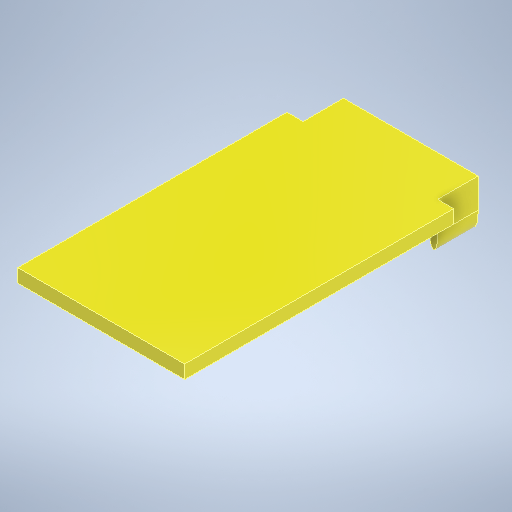
# Autodesk Inventor part: Soporte
Saved by Autodesk Inventor 2025.3 (Build 293356000, 356)
## iProperties
Created: 2025-09-16
Part Number: Soporte
Material: Generic
Document SubType Name: Modeling
Designer: steve
Density: 1 g/cm^3
Appearance: Yellow
Author: steve
Autodesk Inventor part; units mm, degrees
ref_plane "YZ Plane" through (0, 0, 0) normal (1, 0, 0) x (0, 1, 0)
ref_plane "XZ Plane" through (0, 0, 0) normal (0, 1, 0) x (-1, 0, 0)
ref_plane "XY Plane" through (0, 0, 0) normal (0, 0, 1) x (1, 0, 0)
sketch "Sketch1" plane through (0, 0, 0) normal (0, 0, 1) x (1, 0, 0)
  line L0 (-25, 0) -> (25, 0) construction
  line L1 (-25, 25.5) -> (-25, -25.5)
  line L2 (-28, 25.5) -> (-28, -25.5)
  line L3 (0, 25.5) -> (0, -25.5) construction
  line L4 (25, 25.5) -> (25, -25.5)
  line L5 (28, 25.5) -> (28, -25.5)
  line L6 (-25, -25.5) -> (-25, -19.5)
  line L7 (-25, 25.5) -> (-25, 19.5)
  line L8 (-25, 19.5) -> (-25, 26.8474) construction
  line L9 (-25, 26.8474) -> (-22.3693, 26.8474) construction
  line L10 (-22.3693, 26.8474) -> (-18.3013, 21.6592) construction
  spline S0 degree 3 poles (-25, 19.5) (-25, 26.8474) (-22.3693, 26.8474) (-18.3013, 21.6592) knots 1 1 1 1 2 2 2 2
  line L11 (25, 19.5) -> (25, 26.8474) construction
  line L12 (25, 26.8474) -> (22.3693, 26.8474) construction
  line L13 (22.3693, 26.8474) -> (18.3013, 21.6592) construction
  spline S1 degree 3 poles (25, 19.5) (25, 26.8474) (22.3693, 26.8474) (18.3013, 21.6592) knots 1 1 1 1 2 2 2 2
  arc A0 (18.3013, 21.6592) -> (-18.3013, 21.6592) centre (0, -20.023) ccw
  line L14 (-25, -19.5) -> (-25, -27.5122) construction
  line L15 (-25, -27.5122) -> (-22, -27.5122) construction
  line L16 (-22, -27.5122) -> (-22, -19.5) construction
  spline S2 degree 3 poles (-25, -19.5) (-25, -27.5122) (-22, -27.5122) (-22, -19.5) knots 1 1 1 1 2 2 2 2
  line L17 (25, -19.5) -> (25, -27.5122) construction
  line L18 (25, -27.5122) -> (22, -27.5122) construction
  line L19 (22, -27.5122) -> (22, -19.5) construction
  spline S3 degree 3 poles (25, -19.5) (25, -27.5122) (22, -27.5122) (22, -19.5) knots 1 1 1 1 2 2 2 2
  arc A1 (-22, -19.5) -> (22, -19.5) centre (0, 17.8333) ccw
  line L20 (-25, -25.5) -> (-25, -8.5)
  line L21 (-25, -8.5) -> (25, -8.5)
  line L22 (0, -25.5) -> (0, -13.5)
  line L23 (22, -13.5) -> (-22, -13.5)
  line L24 (-22, -19.5) -> (-22, -13.5)
  line L25 (22, -19.5) -> (22, -13.5)
  point P0 (0, 0)
  point P1 (-28, 0)
  point P2 (25, -19.5001)
  dimension "d0" = 50
  dimension "d1" = 3
  dimension "d2" = 51
  dimension "d3" = 3
  dimension "d4" = 51
  dimension "d5" = 51
  dimension "d6" = 0
  dimension "d7" = 6
  dimension "d10" = 6
  dimension "d11" = 3
  dimension "d12" = 17
  dimension "d13" = 12
  constraints: 28 end point, 8 symmetric about line, 7 point on line, 6 midpoint, 6 point on circle, 6 vertical, 2 centre point, 2 horizontal, 2 perpendicular, 1 parallel, 12 other
  measures "d0" distance of L0.start L0.end
  measures "d1" distance between parallel lines of L2 L1
  measures "d2" distance of L3.start L3.end
  measures "d3" distance between parallel lines of L4 L5
  measures "d4" distance of L1.start L1.end
  measures "d5" distance of L2.start L2.end
  measures "d6" vertical distance of point (-28, 0) L0.start
  measures "d7" distance of L1.end L6.end
  measures "d10" distance of L1.start L7.end
  measures "d11" distance of L6.end L16.end
  measures "d12" distance of L1.end L20.end
  measures "d13" distance of L3.end L22.end
extrude "Extrusion1" add sketch "Sketch1" along normal mid plane 15 contours L21 L4 S3 L25 L23 L24 S2 L1
sketch "Sketch3" plane through (0, 0, 7.5) normal (0, 0, 1) x (1, 0, 0)
  line L0 (-25, -8.5) -> (-25, -19.5) projected
  line L1 (25, -8.5) -> (-25, -8.5) projected
  line L2 (25, -19.5001) -> (25, -8.5) projected
  line L3 (-22, -13.5) -> (22, -13.5) projected
  line L4 (22, -13.5) -> (22, -19.5) projected
  line L5 (-22, -19.5) -> (-22, -13.5) projected
  line L6 (-25, -8.5) -> (25, -8.5)
  line L7 (-31, -8.5) -> (31, -8.5)
  line L8 (-31, -8.5) -> (-31, -13.5)
  line L9 (-31, -13.5) -> (31, -13.5)
  line L10 (31, -13.5) -> (31, -8.5)
  point P0 (0, 0)
  point P1 (0, -8.5)
  dimension "d17" = 62
  constraints: 10 end point, 2 midpoint, 2 point on line, 1 horizontal, 1 horizontal alignment, 1 parallel, 1 perpendicular, 1 other
  measures "d17" distance of L7.start L7.end
extrude "Extrusion2" add sketch "Sketch3" along normal blind 100
body "Solid1"
